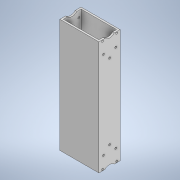
# Autodesk Inventor part: мотор_локтя_2.1-кисти_1
Saved by Autodesk Inventor 2022 (Build 260153000, 153)
## iProperties
Created: 2022-12-04
Part Number: мотор_локтя_2.1-кисти_1
Material: Типовые
Document SubType Name: Modeling
Designer: Папа
Density: 1 g/cm^3
Appearance: По умолчанию
Author: Папа
Autodesk Inventor part; units mm, degrees
ref_plane "YZ Plane" through (0, 0, 0) normal (1, 0, 0) x (0, 1, 0)
ref_plane "XZ Plane" through (0, 0, 0) normal (0, 1, 0) x (-1, 0, 0)
ref_plane "XY Plane" through (0, 0, 0) normal (0, 0, 1) x (1, 0, 0)
sketch "Эскиз2" plane through (0, 0, 0) normal (0, 1, 0) x (-1, 0, 0)
  line L0 (20.1, -10) -> (-20.1, -10)
  line L1 (-20.1, -10) -> (-20.1, 10)
  line L2 (-20.1, 10) -> (20.1, 10)
  line L3 (20.1, 10) -> (20.1, -10)
  line L4 (20.1, -10) -> (-20.1, 10) construction
  line L5 (-20.1, -10) -> (20.1, 10) construction
  line L6 (22.1, 12) -> (-22.1, 12)
  line L7 (-22.1, 12) -> (-22.1, -12)
  line L8 (-22.1, -12) -> (22.1, -12)
  line L9 (22.1, -12) -> (22.1, 12)
  line L10 (22.1, 12) -> (-22.1, -12) construction
  line L11 (-22.1, 12) -> (22.1, -12) construction
  point P0 (0, 0)
  dimension "d5" = 40.2
  dimension "d6" = 20
  dimension "d7" = 2
  dimension "d8" = 2
  constraints: 24 end point, 4 midpoint, 4 parallel, 2 horizontal, 2 perpendicular
  measures "d5" distance of L0.start L0.end
  measures "d6" distance of L0.end L1.end
  measures "d7" distance between parallel lines of L8 L0
  measures "d8" distance between parallel lines of L7 L1
extrude "Выдавливание1" add sketch "Эскиз2" along normal blind 24.75
sketch "Эскиз4" plane through (22.1, 0, 12) normal (1, 0, 0) x (0, 0, -1)
  line L0 (0, 0) -> (24, 0) projected
  line L1 (24, 0) -> (24, 24.75) projected
  line L2 (0, 24.75) -> (24, 24.75) projected
  line L3 (0, 0) -> (0, 24.75) projected
  line L4 (22, 24.75) -> (2, 24.75) projected
  line L5 (12, 24.75) -> (12, 1.55) construction
  line L6 (12, 1.55) -> (20, 1.55) construction
  circle A0 centre (20, 1.55) radius 1.1
  line L7 (12, 14.77) -> (19, 14.77) construction
  circle A1 centre (19, 14.77) radius 1.1
  circle A2 centre (12, 21.77) radius 1.1
  circle A3 centre (4, 1.55) radius 1.1
  line L8 (12, 14.77) -> (5, 14.77) construction
  circle A4 centre (5, 14.77) radius 1.1
  line L9 (12, 1.55) -> (4, 1.55) construction
  point P0 (12, 0)
  dimension "d13" = 23.2
  dimension "d14" = 8
  dimension "d15" = 2.2
  dimension "d16" = 7
  dimension "d17" = 13.22
  dimension "d18" = 7
  constraints: 10 end point, 5 centre point, 4 symmetric about line, 3 coincident, 2 equal radius, 2 horizontal, 2 point on line, 1 midpoint, 1 vertical, 2 other
  measures "d13" distance of L5.start L5.end
  measures "d14" distance of L5.end L6.end
  measures "d15" diameter of A0
  measures "d16" distance of L7.start L7.end
  measures "d17" distance between parallel lines of L6 L7
  measures "d18" distance from line of L7 A2.centre
extrude "Выдавливание3" cut sketch "Эскиз4" against normal blind 2 contours A0 | A1 | A2 | A3 | A4
sketch "Эскиз5" plane through (-22.1, 0, -12) normal (-1, 0, 0) x (0, 0, 1)
  line L0 (0, 0) -> (24, 0) projected
  line L1 (24, 0) -> (24, 24.75) projected
  line L2 (0, 24.75) -> (24, 24.75) projected
  line L3 (0, 0) -> (0, 24.75) projected
  line L4 (24, 24.75) -> (0, 24.75) projected
  line L5 (12, 24.75) -> (12, 5.2772) construction
  circle A0 centre (19.5, 22.16) radius 1.1
  line L6 (19.5, 22.16) -> (12, 22.16) construction
  circle A1 centre (4.5, 22.16) radius 1.1
  circle A2 centre (19.5, 7.16) radius 1.1
  circle A3 centre (4.5, 7.16) radius 1.1
  point P0 (12, 0)
  dimension "d21" = 2.59
  dimension "d22" = 7.5
  dimension "d23" = 2.2
  dimension "d26" = 15
  dimension "d29" = 15
  constraints: 4 centre point, 4 end point, 2 vertical, 1 horizontal, 1 midpoint, 1 perpendicular, 1 point on line, 6 other
  measures "d21" distance from line of L2 L6.start
  measures "d22" distance from line of L5 L6.start
  measures "d23" diameter of A0
  measures "d26" distance of L6.start A1.centre
  measures "d29" distance of L6.start A2.centre
extrude "Выдавливание4" cut sketch "Эскиз5" against normal blind 2 contours A0 | A1 | A2 | A3
sketch "Эскиз3" plane through (0, 24.75, 0) normal (0, 1, 0) x (1, 0, 0)
  line L0 (-22.1, -12) -> (22.1, -12) projected
  line L1 (22.1, -12) -> (-22.1, -12)
  line L2 (-22.1, -12) -> (-22.1, 12)
  line L3 (-22.1, 12) -> (22.1, 12)
  line L4 (22.1, 12) -> (22.1, -12)
  point P0 (0, 0)
  constraints: 8 end point, 2 parallel, 1 horizontal, 1 perpendicular
extrude "Выдавливание2" add sketch "Эскиз3" along normal blind 2
ref_plane "РабПлоскость3" through (-22.1, 26.75, -12) normal (0, 1, 0) x (1, 0, 0)
sketch "Эскиз7" plane through (0, 26.75, 0) normal (0, 1, 0) x (1, 0, 0)
  line L0 (22.1, -12) -> (22.1, 12) projected
  line L1 (-22.1, 12) -> (-22.1, -12) projected
  line L2 (22.1, -12) -> (-22.1, -12)
  line L3 (-22.1, -12) -> (-22.1, 12)
  line L4 (-22.1, 12) -> (22.1, 12)
  line L5 (22.1, 12) -> (22.1, -12)
  point P0 (0, 0)
  constraints: 8 end point, 2 parallel, 1 horizontal, 1 perpendicular
extrude "Выдавливание5" add sketch "Эскиз7" along normal blind 75
ref_plane "РабПлоскость5" through (0, 64.25, 0) normal (0, 1, 0) x (1, 0, 0)
mirror "Зеркальное отражение2" about plane through (0, 64.25, 0) normal (0, 1, 0) of "Выдавливание3", "Выдавливание1", "Выдавливание4", "Выдавливание2"
sketch "Эскиз9" plane through (22.1, 0, 12) normal (1, 0, 0) x (0, 0, -1)
  circle A0 centre (20, 126.95) radius 1.1 construction
  circle A1 centre (4, 126.95) radius 1.1 construction
  circle A2 centre (19, 113.73) radius 1.1 construction
  circle A3 centre (5, 113.73) radius 1.1 construction
  circle A4 centre (12, 106.73) radius 1.1 construction
  circle A5 centre (20, 1.55) radius 1.1 construction
  circle A6 centre (4, 1.55) radius 1.1 construction
  circle A7 centre (19, 14.77) radius 1.1 construction
  circle A8 centre (5, 14.77) radius 1.1 construction
  circle A9 centre (12, 21.77) radius 1.1 construction
  line L0 (0, 0) -> (24, 0) construction
  line L1 (24, 0) -> (24, 128.5) construction
  line L2 (0, 128.5) -> (24, 128.5) construction
  line L3 (0, 0) -> (0, 128.5) construction
  line L4 (0, 0) -> (0, 128.5) construction
  line L5 (0, 64.25) -> (24, 64.25) construction
  circle A10 centre (12, -5.25) radius 7.5
  line L6 (12, -5.25) -> (12, 0) construction
  circle A11 centre (12, 133.75) radius 7.5
  dimension "d46" = 15
  dimension "d47" = 5.25
  constraints: 4 end point, 2 centre point, 2 midpoint, 1 symmetric about line, 1 vertical, 1 other
  measures "d46" diameter of A10
  measures "d47" distance of L6.start L6.end
extrude "Выдавливание6" cut sketch "Эскиз9" against normal up to surface (44.2 mm away)
sketch "Эскиз6" plane through (0, 48, 0) normal (0, 1, 0) x (1, 0, 0)
  line L0 (-12, -22.1) -> (12, -22.1)
  line L1 (12, -22.1) -> (12, 22.1)
  line L2 (12, 22.1) -> (-12, 22.1)
  line L3 (-12, 22.1) -> (-12, -22.1)
  line L4 (-12, -22.1) -> (12, 22.1) construction
  line L5 (12, -22.1) -> (-12, 22.1) construction
  point P0 (0, 0)
  dimension "d35" = 44.2
  dimension "d36" = 24
  constraints: 12 end point, 2 midpoint, 2 parallel, 1 horizontal, 1 perpendicular
  measures "d35" distance of L2.end L0.start
  measures "d36" distance of L0.start L0.end
equation "\"d48\" = d46"
